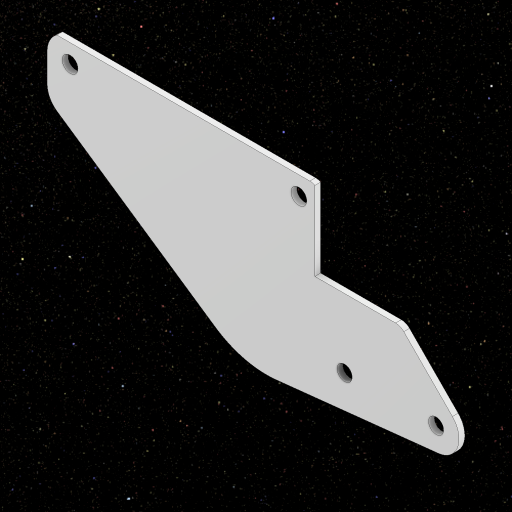
# Autodesk Inventor part: sled
Saved by Autodesk Inventor 2024 (Build 280153000, 153)
## iProperties
Created: 2024-02-11
Part Number: sled
Material: Acetal Resin, White
Document SubType Name: Sheet Metal
Designer: Averey Ku
Density: 1.425 g/cm^3
Appearance: Smooth - White
Flat Pattern Width: 5.2564 cm
Flat Pattern Length: 11.43 cm
Flat Pattern Area: 60.0806 cm^2
Sheet Metal Rule: Default_mm
Sheet Metal Width: 2.069 in
Sheet Metal Length: 4.500 in
Sheet Metal Area: 9.313 in^2
d0: 0.500 in
d1: 0.250 in
d2: 1.000 in
d3: 0.165 in
d4: 0.165 in
d5: 0.172 in
d8: 0.125 in
Author: Averey Ku
Autodesk Inventor part; units mm, degrees
ref_plane "YZ Plane" through (0, 0, 0) normal (1, 0, 0) x (0, 1, 0)
ref_plane "XZ Plane" through (0, 0, 0) normal (0, 1, 0) x (-1, 0, 0)
ref_plane "XY Plane" through (0, 0, 0) normal (0, 0, 1) x (1, 0, 0)
sketch "main" plane through (0, 0, 0) normal (0, 0, 1) x (1, 0, 0)
  arc A0 (7.9061, 59.9189) -> (2.6576, 57.1432) centre (7.9061, 53.5689) ccw
  line L0 (7.9061, 59.9189) -> (15.7951, 59.9189)
  arc A1 (20.9767, 57.2396) -> (15.7951, 59.9189) centre (15.7951, 53.5689) ccw
  circle A2 centre (15.7951, 53.5689) radius 2.1844
  arc A3 (-27.1814, 13.3264) -> (-31.4423, -3.6797) centre (-6.1872, -0.9705) ccw
  circle A4 centre (15.7951, -9.9311) radius 2.1844
  line L1 (20.9767, 57.2396) -> (20.9767, -12.9584)
  circle A5 centre (-20.2983, -22.6311) radius 2.0955
  line L2 (-2.1836, -39.0438) -> (-15.8326, -52.5455)
  circle A6 centre (-20.2983, -48.0311) radius 2.0955
  line L3 (-31.4423, -3.6797) -> (-26.6121, -48.7084)
  arc A7 (-26.6121, -48.7084) -> (-15.8326, -52.5455) centre (-20.2983, -48.0311) ccw
  line L4 (-27.1814, 13.3264) -> (2.6576, 57.1432)
  line L5 (-1.2414, -14.3873) -> (-1.2414, -36.7866)
  arc A8 (20.637, -14.3873) -> (20.9767, -12.9584) centre (17.8017, -12.9584) ccw
  arc A9 (-2.1836, -39.0438) -> (-1.2414, -36.7866) centre (-4.4164, -36.7866) ccw
  line L6 (20.637, -14.3873) -> (-1.2414, -14.3873)
  point P0 (-2.1335, 12.2772)
  point P1 (20.9767, -16.1334)
  dimension "d0" = 12.7
  dimension "d1" = 6.35
  dimension "d2" = 25.4
  dimension "d3" = 4.191
  dimension "d4" = 4.191
  dimension "d5" = 4.3688
  dimension "d8" = 3.175
  measures "d0" diameter of A7
  measures "d1" radius of A0
  measures "d2" radius of A3
  measures "d3" diameter of A5
  measures "d4" diameter of A6
  measures "d5" diameter of A2
  measures "d8" radius of A8
sketch "Sketch1" plane through (0, 0, 0) normal (0, 0, 1) x (1, 0, 0)
  arc A0 (-6.35, -7.889) -> (-3.5742, -13.1375) centre (0, -7.889) ccw
  line L0 (-6.35, -7.889) -> (-6.35, 0)
  arc A1 (-3.6706, 5.1816) -> (-6.35, 0) centre (0, 0) ccw
  circle A2 centre (0, 0) radius 2.1844
  arc A3 (40.2425, -42.9766) -> (57.2486, -47.2375) centre (54.5395, -21.9824) ccw
  circle A4 centre (63.5, 0) radius 2.1844
  line L1 (-3.6706, 5.1816) -> (66.5273, 5.1816)
  circle A5 centre (76.2, -36.0934) radius 2.0955
  line L2 (92.6127, -17.9787) -> (106.1144, -31.6277)
  circle A6 centre (101.6, -36.0934) radius 2.0955
  line L3 (57.2486, -47.2375) -> (102.2773, -42.4072)
  arc A7 (102.2773, -42.4072) -> (106.1144, -31.6277) centre (101.6, -36.0934) ccw
  line L4 (40.2425, -42.9766) -> (-3.5742, -13.1375)
  line L5 (67.9562, -17.0366) -> (90.3555, -17.0366)
  arc A8 (67.9562, 4.8419) -> (66.5273, 5.1816) centre (66.5273, 2.0066) ccw
  arc A9 (92.6127, -17.9787) -> (90.3555, -17.0366) centre (90.3555, -20.2116) ccw
  line L6 (67.9562, 4.8419) -> (67.9562, -17.0366)
  point P0 (0, 0)
  constraints: 1 other
extrude "Extrusion1" add sketch "Sketch1" along normal blind 1.5875
equation "\"BendRadius\" = Thickness"
equation "\"BendReliefWidth\" = Thickness"
equation "\"BendReliefDepth\" = 0.5 * Thickness"
equation "\"CornerReliefSize\" = 4 * Thickness"
equation "\"MinimumRemnant\" = 2 * Thickness"
equation "\"TransitionRadius\" = BendRadius"
equation "\"JacobiRadiusSize\" = BendRadius"
equation "\"GapSize\" = Thickness"
equation "\"Thickness\" = 1.5875"
body "Solid1"
